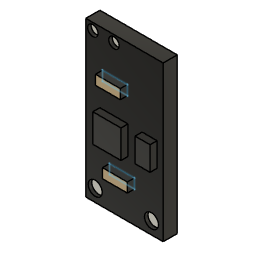
carcasarepetidor (Autodesk Fusion 360 archive; units mm, degrees)
design "DC-DC down"
Autodesk Fusion 360 part; units mm, degrees
sketch "Boceto1" plane through (0, 0, 0) normal (0, 1, 0) x (1, 0, 0)
  line L0 (0, 0) -> (11, 0)
  line L1 (11, 0) -> (11, -22)
  line L2 (11, -22) -> (0, -22)
  line L3 (0, -22) -> (0, 0)
  dimension "d1" = 11
  dimension "d2" = 22
  constraint horizontal L0
  constraint vertical L1
  constraint horizontal L2
  constraint vertical L3
  constraint coincident L0.start L3.end
  measures "d1" distance of L0.start L0.end
  measures "d2" distance of L0.start L2.end
extrude "Extruir1" add sketch "Boceto1" along normal blind 2
sketch "Boceto2" plane through (0, 0, 0) normal (0, -1, 0) x (1, 0, 0)
  line L0 (11, 22) -> (0, 22)
  line L1 (0, 22) -> (0, 0)
  line L2 (0, 0) -> (11, 0)
  line L3 (11, 0) -> (11, 22)
  line L4 (8, 12) -> (10.1306, 12)
  line L5 (10.1306, 12) -> (10.1306, 8.6002)
  line L6 (10.1306, 8.6002) -> (8, 8.6002)
  line L7 (8, 8.6002) -> (8, 12)
  line L8 (2, 12) -> (6, 12)
  line L9 (6, 12) -> (6, 8)
  line L10 (6, 8) -> (2, 8)
  line L11 (2, 8) -> (2, 12)
  constraint horizontal L4
  constraint vertical L5
  constraint horizontal L6
  constraint vertical L7
  constraint horizontal L8
  constraint vertical L9
  constraint horizontal L10
  constraint vertical L11
extrude "Extruir2" add sketch "Boceto2" along normal blind 1 contours L4 L5 L6 L7 | L8 L9 L10 L11
sketch "Boceto3" plane through (0, 0, 0) normal (0, 1, 0) x (1, 0, 0)
  circle A0 centre (1.3364, -1.7459) radius 0.9984
  circle A1 centre (9.3364, -1.7459) radius 0.9984
  circle A2 centre (1, -21) radius 0.7455
  circle A3 centre (4, -21) radius 0.7455
extrude "Extruir3" cut sketch "Boceto3" along normal blind 0.5
sketch "Boceto4" plane through (0, 0, 0) normal (0, 1, 0) x (1, 0, 0)
  line L0 (3.3729, -5.8021) -> (6.9064, -5.8021)
  line L1 (6.9064, -5.8021) -> (6.9064, -4.4369)
  line L2 (6.9064, -4.4369) -> (3.3729, -4.4369)
  line L3 (3.3729, -4.4369) -> (3.3729, -5.8021)
  line L4 (2.3729, -16.8021) -> (5.9064, -16.8021)
  line L5 (5.9064, -15.4369) -> (2.3729, -15.4369)
  line L6 (2.3729, -15.4369) -> (2.3729, -16.8021)
  line L7 (5.9064, -16.8021) -> (5.9064, -15.4369)
  constraint horizontal L0
  constraint vertical L1
  constraint horizontal L2
  constraint vertical L3
  constraint horizontal L4
  constraint vertical L7
  constraint horizontal L5
  constraint vertical L6
extrude "Extruir5" add sketch "Boceto4" against normal blind 1

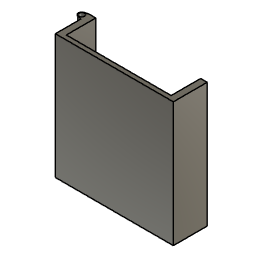
design "carcasarepetidorp2"
Autodesk Fusion 360 part; units mm, degrees
sketch "Boceto1" plane through (0, 0, 0) normal (0, 1, 0) x (1, 0, 0)
  line L0 (0, 0) -> (54, 0)
  line L1 (54, 0) -> (54, -54)
  line L2 (0, -55.5009) -> (0, 0)
  line L3 (3, -55.5009) -> (3, -3)
  line L4 (3, -3) -> (51, -3)
  line L5 (51, -3) -> (51, -54)
  line L6 (51, -54) -> (51, -57)
  line L7 (54, -54) -> (54, -57)
  line L8 (51, -57) -> (54, -57)
  line L9 (3, -55.5009) -> (3, -57)
  line L10 (0, -55.5009) -> (0, -57)
  line L11 (3, -57) -> (0, -57)
  point P0 (52.9294, -57)
  dimension "d1" = 54
  constraint horizontal L0
  constraint vertical L1
  constraint vertical L2
  constraint coincident L0.start L2.end
  constraint perpendicular L0 L3
  constraint perpendicular L1 L4
  constraint perpendicular L4 L5
  constraint parallel L1 L7
  constraint perpendicular L7 L8
  constraint perpendicular L10 L11
  measures "d1" distance of L0.start L0.end
extrude "Extruir1" add sketch "Boceto1" along normal blind 13.5
sketch "Boceto2" plane through (0, 13.5, 0) normal (0, 1, 0) x (-1, 0, 0)
  line L0 (-54, 57) -> (-54, 0)
  line L1 (-54, 0) -> (0, 0)
  line L2 (0, 0) -> (0, 57)
  line L3 (-54, 0) -> (0, 0)
  line L4 (0, 0) -> (0, 57)
  line L5 (0, 57) -> (-54, 57)
  line L6 (-54, 57) -> (-54, 0)
  line L7 (-3, 57) -> (-3, 3)
  line L8 (-3, 3) -> (-51, 3)
  line L9 (-51, 3) -> (-51, 57)
  line L10 (-51, 57) -> (-54, 57)
  line L11 (0, 57) -> (-3, 57)
  constraint horizontal L3
  constraint vertical L4
  constraint horizontal L5
  constraint vertical L6
  constraint coincident L2.end L4.end
  constraint coincident L0.end L1.start
sketch "Boceto3" plane through (0, 0, 0) normal (0, -1, 0) x (1, 0, 0)
  line L0 (0, 57) -> (0, 0)
  line L1 (0, 0) -> (54, 0)
  line L2 (54, 0) -> (54, 57)
  line L3 (51, 57) -> (51, 3)
  line L4 (51, 3) -> (3, 3)
  line L5 (3, 3) -> (3, 57)
  line L6 (0, 0) -> (54, 0)
  line L7 (54, 0) -> (54, 57)
  line L8 (54, 57) -> (0, 57)
  line L9 (0, 57) -> (0, 0)
  line L10 (3, 57) -> (0, 57)
  line L11 (54, 57) -> (51, 57)
  constraint horizontal L6
  constraint vertical L7
  constraint horizontal L8
  constraint vertical L9
  constraint coincident L2.end L7.end
  constraint coincident L0.end L1.start
extrude "Extruir3" add sketch "Boceto3" along normal blind 2
sketch "Boceto4" plane through (0, 0, 57) normal (0, 0, 1) x (-1, 0, 0)
  line L0 (-3, 0) -> (-3, -13.5)
  line L1 (-3, -13.5) -> (0, -13.5)
  line L2 (0, -13.5) -> (0, 2)
  line L3 (0, 2) -> (-54, 2)
  line L4 (-54, 2) -> (-54, -13.5)
  line L5 (-54, -13.5) -> (-51, -13.5)
  line L6 (-51, -13.5) -> (-51, 0)
  line L7 (-51, 0) -> (-3, 0)
  line L8 (-27, 2) -> (-27, -15.6154)
  circle A0 centre (1.5, -11.5767) radius 1.5
  line L9 (0, -13.5) -> (1.8654, -13.0315)
  line L10 (1.5, -11.5767) -> (0.8268, -11.5767)
  line L11 (0, -9.6534) -> (1.8654, -10.1219)
  circle A1 centre (1.5, -11.5767) radius 1.25
  dimension "d10" = 3
  dimension "d11" = 2.5
  constraint midpoint L3 L8.start
  constraint perpendicular L3 L8
  constraint tangent L2 A0
  constraint coincident L1.end L2.start
  constraint coincident A0 L9.end
  constraint tangent A0 L9
  constraint coincident A0.centre L10.start
  constraint perpendicular L2 L10
  constraint symmetric L1.end L10 L11.start
  constraint symmetric L9.end L10 L11.end
  constraint concentric A0 A1
  measures "d10" diameter of A0
  measures "d11" diameter of A1
extrude "Extruir4" add sketch "Boceto4" against normal blind 57 contours L2 A0 L9 | L2 A0 L11 | A0

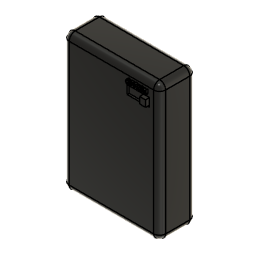
design "Caja Pilas"
Autodesk Fusion 360 part; units mm, degrees
sketch "Sketch1" plane through (0, 0, 0) normal (0, 1, 0) x (1, 0, 0)
  line L0 (0, 0) -> (48, 0)
  line L1 (48, 0) -> (48, -68)
  line L2 (48, -68) -> (0, -68)
  line L3 (0, -68) -> (0, 0)
  dimension "d1" = 48
  dimension "d2" = 68
  constraint horizontal L0
  constraint vertical L1
  constraint horizontal L2
  constraint vertical L3
  constraint coincident L0.start L3.end
  measures "d1" distance of L0.start L0.end
  measures "d2" distance of L0.start L2.end
extrude "Extrude1" add sketch "Sketch1" along normal blind 18
fillet "Fillet1" radius 3 12 edges at (48, 9, 68) (24, 18, 68) (24, 0, 68) (48, 0, 34) (48, 9, 0) (24, 18, 0) (24, 0, 0) (0, 9, 0) (0, 0, 34) (0, 18, 34) (0, 9, 68) (48, 18, 34)
sketch "Boceto2" plane through (0, 0, 0) normal (0, -1, 0) x (1, 0, 0)
  line L0 (45, 65) -> (3, 65)
  line L1 (3, 65) -> (3, 3)
  line L2 (3, 3) -> (45, 3)
  line L3 (45, 3) -> (45, 65)
  line L4 (31.7729, 60.7203) -> (42.8614, 60.7203)
  line L5 (42.8614, 60.7203) -> (42.8614, 56.4555)
  line L6 (42.8614, 56.4555) -> (31.7729, 56.4555)
  line L7 (31.7729, 56.4555) -> (31.7729, 60.7203)
  constraint horizontal L4
  constraint vertical L5
  constraint horizontal L6
  constraint vertical L7
extrude "Extruir2" cut sketch "Boceto2" against normal blind 1 contours L4 L5 L6 L7
sketch "Boceto3" plane through (0, 1, 0) normal (0, -1, 0) x (1, 0, 0)
  line L0 (31.7729, 56.4555) -> (42.8614, 56.4555)
  line L1 (42.8614, 56.4555) -> (42.8614, 60.7203)
  line L2 (42.8614, 60.7203) -> (31.7729, 60.7203)
  line L3 (31.7729, 60.7203) -> (31.7729, 56.4555)
  line L4 (39.5545, 60.2451) -> (42.5, 60.2451)
  line L5 (42.5, 60.2451) -> (42.5, 57)
  line L6 (42.5, 57) -> (39.5545, 57)
  line L7 (39.5545, 57) -> (39.5545, 60.2451)
  constraint horizontal L4
  constraint vertical L5
  constraint horizontal L6
  constraint vertical L7
extrude "Extruir3" add sketch "Boceto3" along normal blind 2.5 contours L4 L5 L6 L7
sketch "Boceto4" plane through (0, 0, 0) normal (0, -1, 0) x (1, 0, 0)
  line L0 (42.8614, 60.7203) -> (42.8614, 56.4555)
  line L1 (42.8614, 56.4555) -> (31.7729, 56.4555)
  line L2 (31.7729, 56.4555) -> (31.7729, 60.7203)
  line L3 (31.7729, 60.7203) -> (42.8614, 60.7203)
  line L4 (45, 65) -> (3, 65)
  line L5 (3, 65) -> (3, 3)
  line L6 (3, 3) -> (45, 3)
  line L7 (45, 3) -> (45, 65)
  line L8 (31.9974, 60.7278) -> (41.3548, 60.7203) construction
  line L9 (41.3548, 60.7203) -> (41.3575, 63.9925) construction
  line L10 (41.3575, 63.9925) -> (32, 64) construction
  line L11 (32, 64) -> (31.9974, 60.7278) construction
  dimension "d11" = 2
  text T0 "OFF/ON" font "Arial" height 2 align left top in box 9.3575 x 3.2722 at (31.9974, 60.7278) x (1, -0.000799) y (0.000799, 1) spacing 1 kerned
  constraint coincident L3
extrude "Extruir4" add sketch "Boceto4" along normal blind 1 text T0

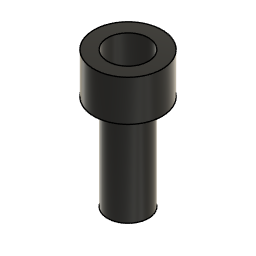
design "TORNILLOM3"
Autodesk Fusion 360 part; units mm, degrees
sketch "Boceto1" plane through (0, 0, 0) normal (0, 0, 1) x (1, 0, 0)
  circle A0 centre (0, 0) radius 1.5
  dimension "d1" = 3
  constraint coincident A0.centre origin
  measures "d1" diameter of A0
extrude "Extruir1" add sketch "Boceto1" along normal blind 7 makes body 1
sketch "Boceto2" plane through (0, 0, 7) normal (0, 0, 1) x (-1, 0, 0)
  circle A0 centre (0, 0) radius 1.5
  circle A1 centre (0, 0) radius 2.5
  dimension "d4" = 5
  constraint concentric A0 A1
  measures "d4" diameter of A1
extrude "Extruir2" add sketch "Boceto2" along normal blind 3 separate body makes body 2
